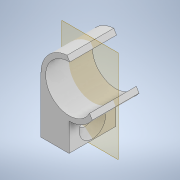
# Autodesk Inventor part: shadeHolderV02
Saved by Autodesk Inventor 2021.2 (Build 252289000, 289)
## iProperties
Created: 2021-02-12
Part Number: shadeHolderV02
Material: Generic
Document SubType Name: Modeling
Designer: robst
Density: 1 g/cm^3
Appearance: Default
Author: robst
Autodesk Inventor part; units mm, degrees
ref_plane "YZ Plane" through (0, 0, 0) normal (1, 0, 0) x (0, 1, 0)
ref_plane "XZ Plane" through (0, 0, 0) normal (0, 1, 0) x (-1, 0, 0)
sketch "Sketch4" plane through (0, 0, 0) normal (0, 0, 1) x (1, 0, 0)
  arc A0 (0.1982, 6.3469) -> (5.5957, -3.0018) centre (0, 0) ccw
  arc A1 (-0.5263, 7.6018) -> (6.3202, -4.2567) centre (0, 0) ccw
  line L0 (0, 0) -> (0, 7.9375) construction
  line L1 (0.1982, 6.3469) -> (5.5957, -3.0018) construction
  line L2 (0.1982, 6.3469) -> (-0.5263, 7.6018)
  line L3 (5.5957, -3.0018) -> (6.3202, -4.2567)
  circle A2 centre (0, 0) radius 6.35
  dimension "d10" = 12.7
  dimension "d11" = 1.27
  dimension "d12" = 30
  dimension "d13" = 10.795
  constraints: 8 end point, 4 point on circle, 3 centre point, 3 coincident, 1 collinear, 1 concentric, 1 point on line, 1 vertical
  measures "d10" diameter of A0
  measures "d11" radial gap between concentric circles of A1 A0
  measures "d12" angle of L1 L0
  measures "d13" distance of L1.start L1.end
extrude "Extrusion3" add sketch "Sketch4" along normal mid plane 12.7 contours A0 L3 A1 L2
sketch "Sketch5" plane through (0, 0, 0) normal (0, 0, 1) x (1, 0, 0)
  arc A0 (-0.5263, 7.6018) -> (6.3202, -4.2567) centre (0, 0) ccw projected
  line L0 (-7.62, 0) -> (-7.62, -15.24)
  line L1 (-7.62, -15.24) -> (0, -15.24)
  line L2 (0, -15.24) -> (0, -7.62)
  circle A1 centre (0, 0) radius 7.9375
  dimension "d16" = 7.62
  constraints: 6 end point, 2 perpendicular, 2 point on circle, 1 centre point, 1 coincident, 1 tangent, 1 vertical
  measures "d16" distance from line of L2.end L1
extrude "Extrusion4" add sketch "Sketch5" along normal mid plane 12.7 contours A0 L2 A1 L0 | A1 L2 L1 L0 picked at (-7.3048, -2.4081)
sketch "Sketch6" plane through (0, -15.24, 6.35) normal (1, 0, 0) x (0, 0, -1)
  line L0 (0, 7.62) -> (12.7, 7.62) projected
  line L1 (12.7, 7.62) -> (12.7, 0) projected
  line L2 (0, 0) -> (12.7, 0) projected
  line L3 (0, 0) -> (0, 7.62) projected
  line L4 (0, 7.62) -> (12.7, 0) construction
  line L5 (12.7, 7.62) -> (0, 0) construction
  point P0 (6.35, 15.24)
  point P1 (6.35, 3.81)
  constraints: 4 end point, 1 midpoint
hole "Hole1" at (0, -11.43, 0) direction (-1, 0, 0) diameter 3.5052 end through all countersink diameter 7.112 countersink angle 82
equation "\"d10\" = shadeDiameter"
equation "\"d11\" = shadeHolderWallThickness"
equation "\"d13\" = openingForShade"
equation "\"d14\" = partWidth"
equation "\"d16\" = flatBelowShade"
equation "\"d17\" = partWidth"
equation "\"shadeDiameter\" = 12.7"
equation "\"partWidth\" = 12.7"
equation "\"backThickness\" = 1.905"
equation "\"backHeight\" = 25.4"
equation "\"cutTiltAngle\" = 60deg"
equation "\"flatBelowShade\" = 7.62"
equation "\"shadeHolderWallThickness\" = 1.27"
equation "\"openingForShade\" = 10.795"
body "Solid2"
